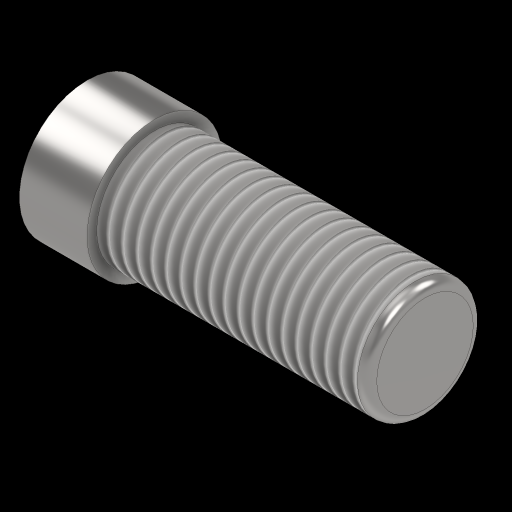
# Autodesk Inventor part: bolt
Saved by Autodesk Inventor 2024 (Build 280153000, 153)
## iProperties
Created: 2023-10-30
Part Number: bolt
Material: Steel, Cast
Document SubType Name: Modeling
Designer: Admin
Density: 7.85 g/cm^3
Appearance: Semi-Polished
Author: Admin
Autodesk Inventor part; units mm, degrees
ref_plane "YZ Plane" through (0, 0, 0) normal (1, 0, 0) x (0, 1, 0)
ref_plane "XZ Plane" through (0, 0, 0) normal (0, 1, 0) x (-1, 0, 0)
ref_plane "XY Plane" through (0, 0, 0) normal (0, 0, 1) x (1, 0, 0)
sketch "Sketch2" plane through (0, 0, 0) normal (1, 0, 0) x (0, 1, 0)
  circle A0 centre (0, 0) radius 7
  circle A1 centre (0, 0) radius 6
  dimension "d0" = 14
  dimension "d1" = 12
  constraints: 2 centre point, 2 coincident
  measures "d0" diameter of A0
  measures "d1" diameter of A1
extrude "Extrusion1" add sketch "Sketch2" along normal blind 35 contours A1
extrude "Extrusion2" add sketch "Sketch2" along normal blind 7 contours A0 | A1
fillet "Fillet1" radius 1 1 edges at (35, -6, 0)
thread "Thread1" size "M12x1.5" class "6g" standard "ANSI Metric M Profile" length 30
body "Solid1"
